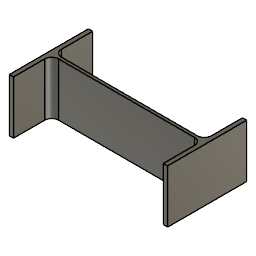
H-298×149×5×8 (Autodesk Fusion 360 design; units mm, degrees)
Autodesk Fusion 360 part; units mm, degrees
sketch "スケッチ1" plane through (0, 0, 0) normal (0, 0, 1) x (1, 0, 0)
  line L0 (0, 74.5) -> (0, -74.5)
  line L1 (298, -74.5) -> (298, 74.5)
  line L2 (290, -15.75) -> (290, -74.5)
  line L3 (8, -74.5) -> (8, -15.75)
  line L4 (0, -74.5) -> (8, -74.5)
  line L5 (290, -74.5) -> (298, -74.5)
  line L6 (277, 2.75) -> (21, 2.75)
  line L7 (21, -2.75) -> (277, -2.75)
  line L8 (8, 15.75) -> (8, 74.5)
  arc A0 (8, 15.75) -> (21, 2.75) centre (21, 15.75) ccw
  arc A1 (21, -2.75) -> (8, -15.75) centre (21, -15.75) ccw
  line L9 (8, 74.5) -> (0, 74.5)
  line L10 (290, 74.5) -> (290, 15.75)
  arc A2 (277, 2.75) -> (290, 15.75) centre (277, 15.75) ccw
  arc A3 (290, -15.75) -> (277, -2.75) centre (277, -15.75) ccw
  line L11 (298, 74.5) -> (290, 74.5)
extrude "押し出し1" add sketch "スケッチ1" along normal blind 100
